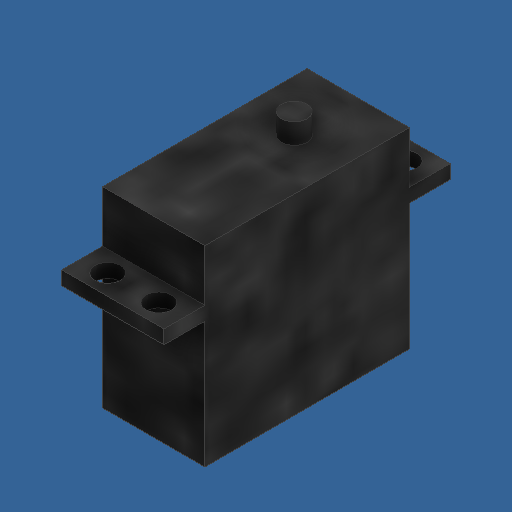
# Autodesk Inventor part: motor
Saved by Autodesk Inventor 2025 (Build 290162000, 162)
## iProperties
Created: 2024-11-29
Part Number: motor
Material: Generic
Document SubType Name: Modeling
Designer: Pauline Simonnet
Density: 1 g/cm^3
Appearance: Asphalt 2
Author: Pauline Simonnet
Autodesk Inventor part; units mm, degrees
ref_plane "YZ Plane" through (0, 0, 0) normal (1, 0, 0) x (0, 1, 0)
ref_plane "XZ Plane" through (0, 0, 0) normal (0, 1, 0) x (-1, 0, 0)
ref_plane "XY Plane" through (0, 0, 0) normal (0, 0, 1) x (1, 0, 0)
sketch "Sketch1" plane through (0, 0, 0) normal (0, 1, 0) x (-1, 0, 0)
  line L0 (0, 0) -> (20, 0)
  line L1 (20, 0) -> (20, -40)
  line L2 (20, -40) -> (0, -40)
  line L3 (0, -40) -> (0, 0)
  dimension "d0" = 40
  dimension "d1" = 20
  constraints: 8 end point, 2 parallel, 1 horizontal, 1 perpendicular
  measures "d0" distance of L0.end L1.end
  measures "d1" distance of L1.end L2.end
extrude "Extrusion1" add sketch "Sketch1" along normal blind 24.7
sketch "Sketch2" plane through (0, 24.7, 0) normal (0, 1, 0) x (1, 0, 0)
  line L0 (0, -8) -> (-20, -8)
  line L1 (-20, -8) -> (-20, 48)
  line L2 (-20, 48) -> (0, 48)
  line L3 (0, 48) -> (0, -8)
  line L4 (-20, 40) -> (-20, 0) projected
  line L5 (-20, 0) -> (0, 0) projected
  dimension "d4" = 56
  dimension "d5" = 20
  dimension "d6" = 0
  dimension "d7" = 8
  constraints: 8 end point, 2 parallel, 1 horizontal, 1 perpendicular
  measures "d4" distance of L0.end L1.end
  measures "d5" distance of L0.start L0.end
  measures "d6" distance between parallel lines of L4 L1
  measures "d7" distance between parallel lines of L5 L0
extrude "Extrusion2" add sketch "Sketch2" along normal blind 2.7
sketch "Sketch3" plane through (0, 27.4, 0) normal (0, 1, 0) x (1, 0, 0)
  line L0 (-20, 48) -> (-20, 40) projected
  line L1 (0, 0) -> (-20, 0)
  line L2 (-20, 0) -> (-20, 40)
  line L3 (-20, 40) -> (0, 40)
  line L4 (0, 40) -> (0, 0)
  constraints: 8 end point, 2 parallel, 1 horizontal, 1 perpendicular
extrude "Extrusion3" add sketch "Sketch3" along normal blind 10.1
sketch "Sketch4" plane through (0, 37.5, 0) normal (0, 1, 0) x (1, 0, 0)
  circle A0 centre (-10, 27.5) radius 2.5
  line L0 (0, 40) -> (-20, 40) projected
  line L1 (0, 0) -> (0, 40) projected
  dimension "d12" = 12.5
  dimension "d13" = 5
  dimension "d16" = 10
  constraints: 1 centre point
  measures "d12" distance from line of L0 A0.centre
  measures "d13" diameter of A0
  measures "d16" distance from line of L1 A0.centre
extrude "Extrusion4" add sketch "Sketch4" along normal blind 4
sketch "Sketch5" plane through (0, 27.4, 0) normal (0, 1, 0) x (1, 0, 0)
  circle A0 centre (-5, -4) radius 2.5
  circle A1 centre (-15, -4) radius 2.5
  line L0 (-20, 0) -> (-20, -8) projected
  line L1 (0, -8) -> (0, 0) projected
  line L2 (-20, -8) -> (0, -8) projected
  line L3 (17.0621, 20) -> (-50.3662, 20) construction
  line L4 (-20, 0) -> (0, 0) projected
  circle A2 centre (-5, 44) radius 2.5
  circle A3 centre (-15, 44) radius 2.5
  dimension "d17" = 5
  dimension "d18" = 5
  dimension "d19" = 5
  dimension "d20" = 4
  dimension "d21" = 4
  dimension "d22" = 20
  constraints: 4 centre point, 2 end point, 2 symmetric about line, 1 equal radius, 1 horizontal, 2 other
  measures "d17" diameter of A1
  measures "d18" distance from line of L0 A1.centre
  measures "d19" distance from line of A0.centre L1
  measures "d20" distance from line of L2 A0.centre
  measures "d21" distance from line of L2 A1.centre
  measures "d22" distance between parallel lines of L4 L3
extrude "Extrusion5" cut sketch "Sketch5" against normal blind 4 contours A0 | A1 | A2 | A3
equation "\"d21\" = d20"
body "Solid1"
